4cf86f36-a587-4e07-97b9-b429af0fc345 (Autodesk Fusion 360 design; units mm, degrees)
Autodesk Fusion 360 part; units mm, degrees
note: some values were not read from the file. Set by a fixed rule: which sketch regions a step uses.
sketch "Sketch1" plane through (0, 0, 0) normal (0, 1, 0) x (1, 0, 0)
  circle A0 centre (0, 0) radius 7.62
  circle A1 centre (0, 0) radius 8.89
  circle A2 centre (0, 0) radius 6.35
  circle A3 centre (0, 0) radius 7.1605
  arc A4 (8.8672, -0.636) -> (-8.1484, -3.5548) centre (0, 0) ccw
  circle A5 centre (0, 0) radius 3.9688
  line L0 (0, 0) -> (8.89, 0) construction
  line L1 (0, 0) -> (-0.6241, -7.1332)
  line L2 (0, 0) -> (-1.2434, -7.0517)
  line L3 (0, 0) -> (-1.8533, -6.9165)
  line L4 (0, 0) -> (-2.449, -6.7286)
  line L5 (0, 0) -> (-3.0261, -6.4896)
  line L6 (0, 0) -> (-3.5802, -6.2011)
  line L7 (0, 0) -> (-4.1071, -5.8655)
  line L8 (-0.6241, -7.1332) -> (-0.0016, -7.1877) construction
  line L9 (-1.2434, -7.0517) -> (-0.0127, -7.2687) construction
  line L10 (-1.8533, -6.9165) -> (-0.0425, -7.4017) construction
  line L11 (-2.449, -6.7286) -> (-0.1003, -7.5835) construction
  line L12 (-3.0261, -6.4896) -> (-0.1945, -7.81) construction
  line L13 (-3.5802, -6.2011) -> (-0.3333, -8.0757) construction
  line L14 (-4.1071, -5.8655) -> (-0.524, -8.3744) construction
  line L15 (0, 0) -> (-4.6027, -5.4852)
  line L16 (-4.6027, -5.4852) -> (-0.7732, -8.6985) construction
  line L17 (0, 0) -> (-5.0632, -5.0632)
  line L18 (-5.0632, -5.0632) -> (-1.0866, -9.0398) construction
  spline S0 degree 5 poles (-1.0866, -9.0398) (-1.0757, -9.0281) (-1.0541, -9.0049) (-1.0218, -8.9702) (-0.9791, -8.9247) (-0.9266, -8.8687) (-0.8752, -8.8132) (-0.8251, -8.758) (-0.7765, -8.7028) (-0.7296, -8.6474) (-0.6844, -8.5918) (-0.641, -8.5361) (-0.5993, -8.4803) (-0.5591, -8.4248) (-0.5204, -8.3696) (-0.4832, -8.3148) (-0.4473, -8.2607) (-0.4128, -8.2071) (-0.3798, -8.1542) (-0.3483, -8.1018) (-0.3182, -8.05) (-0.2897, -7.9988) (-0.2627, -7.9483) (-0.2372, -7.8986) (-0.2131, -7.8497) (-0.1905, -7.8018) (-0.1692, -7.7549) (-0.1494, -7.7091) (-0.1309, -7.6644) (-0.1139, -7.6208) (-0.0983, -7.5785) (-0.084, -7.5375) (-0.071, -7.4979) (-0.0592, -7.46) (-0.0486, -7.4238) (-0.0391, -7.3895) (-0.0307, -7.357) (-0.0235, -7.3265) (-0.0175, -7.2978) (-0.0128, -7.271) (-0.0092, -7.2463) (-0.0064, -7.2242) (-0.0041, -7.2053) (-0.002, -7.1898) (-0.0001, -7.1781) (0.0014, -7.1697) (0.0017, -7.165) (0.0011, -7.1624) (0.0004, -7.1611) (0, -7.1605) knots 0 0 0 0 0 0 0.022222 0.044444 0.066667 0.088889 0.111111 0.133333 0.155556 0.177778 0.2 0.222222 0.244444 0.266667 0.288889 0.311111 0.333333 0.355556 0.377778 0.4 0.422222 0.444444 0.466667 0.488889 0.511111 0.533333 0.555556 0.577778 0.6 0.622222 0.644444 0.666667 0.688889 0.711111 0.733333 0.755556 0.777778 0.8 0.822222 0.844444 0.866667 0.888889 0.911111 0.933333 0.955556 0.977778 1 1 1 1 1 1
  line L19 (-1.1925, -9.154) -> (-0.9807, -8.9257)
  line L20 (0.0407, -7.2161) -> (-0.0407, -7.1048)
  line L21 (-0.1135, -7.6192) -> (0, 0)
  line L22 (0, 0) -> (-0.8938, -6.0873) construction
  line L23 (0, -7.1605) -> (0, 0) construction
  spline S1 degree 5 poles (0, -7.1605) (0, -7.1058) (0, -7.0063) (0, -6.8865) (0, -6.7746) (0, -6.6686) (0, -6.572) (0, -6.4737) (0, -6.3937) (0, -6.35) knots 0 0 0 0 0 0 0.2 0.4 0.6 0.8 1 1 1 1 1 1
  spline S2 degree 5 poles (-2.0585, -6.8582) (-2.0428, -6.8059) (-2.0142, -6.7106) (-1.9797, -6.5958) (-1.9475, -6.4886) (-1.9171, -6.3871) (-1.8893, -6.2946) (-1.8611, -6.2005) (-1.838, -6.1238) (-1.8255, -6.082) knots 0 0 0 0 0 0 0.2 0.4 0.6 0.8 1 1 1 1 1 1
  line L24 (0, -7.2476) -> (0, -7.0734)
  line L25 (0, -6.4196) -> (0, -6.2804)
  line L26 (-2.0835, -6.9416) -> (-2.0334, -6.7748)
  line L27 (-1.8455, -6.1486) -> (-1.8055, -6.0153)
  spline S3 degree 5 poles (-1.558, -8.9706) (-1.5651, -8.9563) (-1.5791, -8.9278) (-1.6001, -8.8853) (-1.6279, -8.8295) (-1.662, -8.7607) (-1.6953, -8.6928) (-1.7275, -8.6255) (-1.7581, -8.5586) (-1.7872, -8.4921) (-1.8144, -8.4259) (-1.84, -8.36) (-1.8639, -8.2946) (-1.8864, -8.2299) (-1.9076, -8.1659) (-1.9275, -8.1028) (-1.9463, -8.0406) (-1.9639, -7.9794) (-1.9803, -7.9191) (-1.9955, -7.8599) (-2.0094, -7.8017) (-2.022, -7.7444) (-2.0333, -7.6883) (-2.0435, -7.6333) (-2.0525, -7.5796) (-2.0604, -7.5272) (-2.0673, -7.4762) (-2.0731, -7.4266) (-2.0779, -7.3785) (-2.0817, -7.3319) (-2.0845, -7.2868) (-2.0864, -7.2434) (-2.0875, -7.2018) (-2.0879, -7.1621) (-2.0876, -7.1244) (-2.0869, -7.0888) (-2.0856, -7.0553) (-2.0837, -7.024) (-2.0811, -6.9947) (-2.0779, -6.9677) (-2.0743, -6.9431) (-2.0706, -6.9211) (-2.0674, -6.9023) (-2.065, -6.8869) (-2.0635, -6.8751) (-2.0624, -6.8666) (-2.0614, -6.8621) (-2.0601, -6.8598) (-2.0591, -6.8586) (-2.0585, -6.8582) knots 0 0 0 0 0 0 0.022222 0.044444 0.066667 0.088889 0.111111 0.133333 0.155556 0.177778 0.2 0.222222 0.244444 0.266667 0.288889 0.311111 0.333333 0.355556 0.377778 0.4 0.422222 0.444444 0.466667 0.488889 0.511111 0.533333 0.555556 0.577778 0.6 0.622222 0.644444 0.666667 0.688889 0.711111 0.733333 0.755556 0.777778 0.8 0.822222 0.844444 0.866667 0.888889 0.911111 0.933333 0.955556 0.977778 1 1 1 1 1 1
  line L28 (-1.4894, -9.1104) -> (-1.6267, -8.8308)
  line L29 (-2.1134, -6.8998) -> (-2.0035, -6.8166)
  point P0 (-0.1135, -7.6192)
  point P1 (0, -6.35)
  point P2 (-1.76, -8.5536)
  point P3 (-1.9055, -8.1715)
  point P4 (-2.0023, -7.8307)
  point P5 (-2.0589, -7.5362)
  point P6 (-2.084, -7.2922)
  point P7 (-2.0871, -7.1014)
  point P8 (-2.0775, -6.9655)
  point P9 (-2.0648, -6.8847)
  point P10 (-1.8255, -6.082)
  dimension "d2" = 17.78
  dimension "id" = 12.7
  dimension "BaseDiameter" = 14.3209
  dimension "d1" = 7.9375
  dimension "d34" = 5
  dimension "d35" = 5
  dimension "d36" = 5
  dimension "d37" = 5
  dimension "d38" = 5
  dimension "d39" = 5
  dimension "d41" = 0.6249
  dimension "d42" = 1.2497
  dimension "d43" = 1.8746
  dimension "d44" = 2.4995
  dimension "d45" = 3.1243
  dimension "d46" = 3.7492
  dimension "d47" = 4.3741
  dimension "d48" = 5
  dimension "d49" = 4.9989
  dimension "d50" = 5
  dimension "d51" = 5.6238
  dimension "d55" = 7.5
  dimension "d60" = 5
  constraint coincident A0.centre A1.centre
  constraint concentric A0 A2
  constraint coincident A1 A4.end
  constraint horizontal L0
  constraint coincident A4 L0.end
  constraint coincident A3 S0.end
  constraint coincident A3 L1.end
  constraint coincident A3 L2.end
  constraint coincident A3 L3.end
  constraint coincident A3 L4.end
  constraint coincident A3 L5.end
  constraint coincident A3 L6.end
  constraint coincident A3 L7.end
  constraint vertical A0.centre S0.end
  constraint tangent A3 L8
  constraint tangent A3 L9
  constraint tangent A3 L10
  constraint tangent A3 L11
  constraint tangent A3 L12
  constraint tangent A3 L13
  constraint tangent A3 L14
  constraint coincident A3 L15.end
  constraint tangent A3 L16
  constraint coincident A3 L17.end
  constraint tangent A3 L18
  constraint midpoint L18.end L19
  constraint midpoint S0.end L20
  constraint coincident A0 P0
  constraint coincident S0 P0
  constraint coincident P0 L21.start
  constraint coincident L23 P1
  constraint coincident A2 P1
  constraint coincident P1 S1.end
  constraint midpoint S0.end L24
  constraint midpoint P1 L25
  constraint symmetric S0.end L22 S2.start
  constraint symmetric L8.end L22 P9
  constraint symmetric L9.end L22 P8
  constraint symmetric L10.end L22 P7
  constraint symmetric L11.end L22 P6
  constraint symmetric L12.end L22 P5
  constraint symmetric L13.end L22 P4
  constraint symmetric L14.end L22 P3
  constraint symmetric L16.end L22 P2
  constraint symmetric L18.end L22 S3.start
  constraint symmetric L19.start L22 L28.start
  constraint symmetric L19.end L22 L28.end
  constraint symmetric L20.start L22 L29.start
  constraint symmetric L20.end L22 L29.end
  constraint symmetric L22 P1 P10
  constraint symmetric L22 L24.start L26.start
  constraint symmetric L22 L24.end L26.end
  constraint symmetric L22 L25.start L27.start
  constraint symmetric L22 L25.end L27.end
  constraint vertical L24
  constraint vertical L25
  measures "d2" diameter of A1
  measures "id" diameter of A2
  measures "BaseDiameter" diameter of A3
  measures "d1" diameter of A5
  measures "d34" angle of L1 L2
  measures "d35" angle of L2 L3
  measures "d36" angle of L3 L4
  measures "d37" angle of L4 L5
  measures "d38" angle of L5 L6
  measures "d39" angle of L6 L7
  measures "d41" distance of L1.end L8.end
  measures "d42" distance of L2.end L9.end
  measures "d43" distance of L3.end L10.end
  measures "d44" distance of L4.end L11.end
  measures "d45" distance of L5.end L12.end
  measures "d46" distance of L6.end L13.end
  measures "d47" distance of L7.end L14.end
  measures "d48" angle of L7 L15
  measures "d49" distance of L15.end L16.end
  measures "d50" angle of L15 L17
  measures "d51" distance of L17.end L18.end
  measures "d55" angle of L21 L22
  measures "d60" angle of L1 L23
extrude "Extrude1" add sketch "Sketch1" along normal blind 304.8 contours A0 A1 S0 S3 | A3 S0 L21 | A0 A3 L21 S3 | A2 A3 L21 S1 L24 L25 | A2 A3 L1 L21 | A2 A3 L3 S2 L26 L27 | A2 A3 L1 L2 | A2 A3 L2 L3 makes body 1
pattern_circular "C-Pattern2" count 12 over 360 about axis through (0, 1.75, 0) along (0, 1, 0) of bodies 1 makes body 2 at (2.9952, 203.2, 5.5992) makes body 3 at (5.3935, 203.2, 3.3515) makes body 4 at (6.3467, 203.2, 0.2057) makes body 5 at (5.5992, 203.2, -2.9952) makes body 6 at (3.3515, 203.2, -5.3935) makes body 7 at (0.2057, 203.2, -6.3467) makes body 8 at (-2.9952, 203.2, -5.5992) makes body 9 at (-5.3935, 203.2, -3.3515) makes body 10 at (-6.3467, 203.2, -0.2057) makes body 11 at (-5.5992, 203.2, 2.9952) makes body 12 at (-3.3515, 203.2, 5.3935)
extrude "Extrude2" add sketch "Sketch1" along normal blind 304.8 contours A2 A5 L17 L21 | A2 A5 L1 L21 | A2 A5 L1 L2 | A2 A5 L3 L4 | A2 A5 L4 L5 | A2 A5 L2 L3 | A2 A5 L15 L17 | A2 A5 L5 L6 | A2 A5 L7 L15 | A2 A5 L6 L7 bodies 1 2 3 4 5 6 7 8 9 10 11 12
ref_plane "WorkPlane1" through (6.2747, 152.4, -0.8261) normal (0.130526, 0, 0.991445) x (0.991445, 0, -0.130526)
fillet "Fillet1" [suppressed]
mirror "Mirror3" [suppressed]
pattern_circular "C-Pattern1" [suppressed]
equation "d = 0.6 in"
equation "OutsideDiameter = d2"
equation "PitchDiameter = d"
equation "id = PitchDiameter - 2 * ( PitchDiameter / TeethNumber )"
equation "BaseDiameter = PitchDiameter * cos(20 deg)"
equation "Length = 12 in"
equation "t = 12"
equation "ShaftDiameter = d1"
equation "TeethNumber = t"
equation "Pitch = 32"
equation "d30 = ( 1.25 * ( PitchDiameter / TeethNumber ) ) - ( PitchDiameter / TeethNumber )"
equation "Basecircum = PI * PitchDiameter * cos(20 deg)"
equation "d41 = Basecircum * 5 / 360"
equation "d42 = Basecircum * 10 / 360"
equation "d43 = Basecircum * 15 / 360"
equation "d44 = Basecircum * 20 / 360"
equation "d45 = Basecircum * 25 / 360"
equation "d46 = Basecircum * 30 / 360"
equation "d47 = Basecircum * 35 / 360"
equation "d49 = Basecircum * 40 / 360"
equation "d51 = Basecircum * 45 / 360"
equation "d55 = ( 360 / ( 4 * TeethNumber ) ) * 1 deg"
